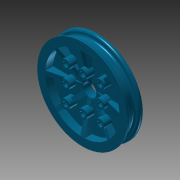
# Autodesk Inventor part: 13-0001
Saved by Autodesk Inventor 2015 SP1 (Build 190203100, 203)
## iProperties
Category: Matrix
Company: Autodesk Inc.
Created: 2014-11-30
Part Number: 13-0001
Material: Polystyrene, High Impact
Document SubType Name: Modeling
Designer: Matrix
Density: 1.022 g/cm^3
Appearance: Sky Blue Dark
Catalog Web Link: http://matrixrobotics.com/
Vendor: Matrix
Author: Autodesk Inc.
Autodesk Inventor part; units mm, degrees
ref_plane "YZ Plane" through (0, 0, 0) normal (1, 0, 0) x (0, 1, 0)
ref_plane "XZ Plane" through (0, 0, 0) normal (0, 1, 0) x (-1, 0, 0)
ref_plane "XY Plane" through (0, 0, 0) normal (0, 0, 1) x (1, 0, 0)
sketch "Sketch1" plane through (0, 0, 0) normal (0, 1, 0) x (-1, 0, 0)
  circle A0 centre (0, 16) radius 2.3444
  circle A1 centre (16, 16) radius 2.3444
  arc A2 (34.4298, 2.2) -> (25.7684, 22.9399) centre (0, 0) ccw
  line L0 (25.7684, 22.9399) -> (25.7597, 22.9313)
  line L1 (25.7597, 22.9313) -> (22.7899, 25.9012)
  arc A3 (22.7899, 25.9012) -> (2, 34.442) centre (0, 0) ccw
  line L2 (2, 34.442) -> (2, 34.4298)
  line L3 (2, 34.4298) -> (-2.2, 34.4298)
  arc A4 (-2.2, 34.4298) -> (-22.9399, 25.7684) centre (0, 0) ccw
  line L4 (-22.9399, 25.7684) -> (-22.9313, 25.7597)
  line L5 (-22.9313, 25.7597) -> (-25.9012, 22.7899)
  arc A5 (-25.9012, 22.7899) -> (-34.442, 2) centre (0, 0) ccw
  line L6 (-34.442, 2) -> (-34.4298, 2)
  line L7 (-34.4298, 2) -> (-34.4298, -2.2)
  arc A6 (-34.4298, -2.2) -> (-25.7684, -22.9399) centre (0, 0) ccw
  line L8 (-25.7684, -22.9399) -> (-25.7597, -22.9313)
  line L9 (-25.7597, -22.9313) -> (-22.7899, -25.9012)
  arc A7 (-22.7899, -25.9012) -> (-2, -34.442) centre (0, 0) ccw
  line L10 (-2, -34.442) -> (-2, -34.4298)
  line L11 (-2, -34.4298) -> (2.2, -34.4298)
  arc A8 (2.2, -34.4298) -> (22.9399, -25.7684) centre (0, 0) ccw
  line L12 (22.9399, -25.7684) -> (22.9313, -25.7597)
  line L13 (22.9313, -25.7597) -> (25.9012, -22.7899)
  arc A9 (25.9012, -22.7899) -> (34.442, -2) centre (0, 0) ccw
  line L14 (34.442, -2) -> (34.4298, -2)
  line L15 (34.4298, -2) -> (34.4298, 2.2)
  circle A10 centre (16, -16) radius 4.265
  circle A11 centre (16, 16) radius 4.265
  circle A12 centre (16, 0) radius 4.265
  circle A13 centre (0, 16) radius 4.265
  circle A14 centre (0, 0) radius 42
  circle A15 centre (0, -16) radius 2.3444
  circle A16 centre (16, -16) radius 2.3444
  circle A17 centre (16, 0) radius 2.3444
  circle A18 centre (-16, 0) radius 4.265
  circle A19 centre (0, -16) radius 4.265
  circle A20 centre (-16, -16) radius 4.265
  circle A21 centre (-16, 16) radius 4.265
  circle A22 centre (-16, -16) radius 2.3444
  circle A23 centre (-16, 0) radius 2.3444
  circle A24 centre (-16, 16) radius 2.3444
  point P0 (0, 0)
  point P1 (0, 0)
  constraints: 32 end point, 25 centre point, 16 point on circle
extrude "Extrusion1" add sketch "Sketch1" along normal blind 14 contours L15 L14 A9 L13 L12 A8 L11 L10 A7 L9 L8 A6 L7 L6 A5 L5 L4 A4 L3 L2 A3 L1 L0 A2 | A10 | A11 | A12 | A13 | A14 | A18 | A19 | A20 | A21
sketch "Sketch2" plane through (0, 0, 0) normal (1, 0, 0) x (0, 1, 0)
  line L0 (14, -13.6556) -> (0, -13.6556) projected
  line L1 (0, -13.6556) -> (0, 13.6556) projected
  line L2 (0, 13.6556) -> (14, 13.6556) projected
  line L3 (14, 13.6556) -> (14, -13.6556) projected
  line L4 (14, -42) -> (0, -42) projected
  line L5 (0, -42) -> (0, -18.3444) projected
  line L6 (0, -18.3444) -> (14, -18.3444) projected
  line L7 (14, -18.3444) -> (14, -42) projected
  line L8 (0, 42) -> (14, 42) projected
  line L9 (14, 42) -> (14, 18.3444) projected
  line L10 (14, 18.3444) -> (0, 18.3444) projected
  line L11 (0, 18.3444) -> (0, 42) projected
  line L12 (0, 42) -> (1, 42)
  arc A0 (3, 40) -> (1, 42) centre (1, 40) ccw
  line L13 (3, 40) -> (3, 39.5)
  arc A1 (3, 39.5) -> (5, 37.5) centre (5, 39.5) ccw
  line L14 (5, 37.5) -> (9, 37.5)
  arc A2 (9, 37.5) -> (11, 39.5) centre (9, 39.5) ccw
  line L15 (11, 39.5) -> (11, 40)
  arc A3 (13, 42) -> (11, 40) centre (13, 40) ccw
  line L16 (13, 42) -> (14, 42)
  line L17 (14, 42) -> (14, 40)
  line L18 (14, 40) -> (13, 39.9913)
  line L19 (13, 39.9913) -> (13, 39.0087)
  line L20 (13, 39.0087) -> (14, 39)
  line L21 (14, 39) -> (14, 37.0133)
  line L22 (1, 42) -> (13, 42)
  line L23 (14, 40) -> (14, 39)
  line L24 (-2.8, 0) -> (16.8, 0) projected
  point P0 (0, 0)
  constraints: 24 end point, 8 point on circle, 4 centre point, 1 collinear, 1 vertical
revolve "Revolution1" cut sketch "Sketch2" angle 360 about axis through (0, -10, 0) along (0, 1, 0) contours L8 A3 L15 A2 L14 A1 L13 A0 | L9 L20 L19 L18
sketch "Sketch3" plane through (0, 14, 0) normal (0, 1, 0) x (1, 0, 0)
  arc A0 (-24.8311, -28.7649) -> (-2.7753, -37.8985) centre (0, 0) ccw
  line L0 (-2.7753, -37.8985) -> (-2.7753, -6.7092)
  line L1 (-2.7753, -6.7092) -> (-24.8311, -28.7649)
  line L2 (14.3804, 14.6632) -> (4.8177, 5.1006)
  line L3 (4.8177, 5.1006) -> (5.1006, 4.8177)
  line L4 (5.1006, 4.8177) -> (14.6632, 14.3804)
  arc A1 (14.6632, 14.3804) -> (15.1927, 14.0614) centre (16, 16) ccw
  line L5 (15.1927, 14.0614) -> (5.5248, 4.3934)
  line L6 (5.5248, 4.3934) -> (5.8077, 4.1106)
  line L7 (5.8077, 4.1106) -> (15.6299, 13.9329)
  arc A2 (15.6299, 13.9329) -> (18.0671, 16.3701) centre (16, 16) ccw
  line L8 (18.0671, 16.3701) -> (27.0209, 25.3238)
  line L9 (27.0209, 25.3238) -> (26.738, 25.6066)
  line L10 (26.738, 25.6066) -> (17.9386, 16.8073)
  arc A3 (17.9386, 16.8073) -> (17.6196, 17.3368) centre (16, 16) ccw
  line L11 (17.6196, 17.3368) -> (26.3138, 26.0309)
  line L12 (26.3138, 26.0309) -> (26.0309, 26.3138)
  line L13 (26.0309, 26.3138) -> (17.3368, 17.6196)
  arc A4 (17.3368, 17.6196) -> (16.8073, 17.9386) centre (16, 16) ccw
  line L14 (16.8073, 17.9386) -> (25.6066, 26.738)
  line L15 (25.6066, 26.738) -> (25.3238, 27.0209)
  line L16 (25.3238, 27.0209) -> (16.3701, 18.0671)
  arc A5 (16.3701, 18.0671) -> (13.9329, 15.6299) centre (16, 16) ccw
  line L17 (13.9329, 15.6299) -> (4.1106, 5.8077)
  line L18 (4.1106, 5.8077) -> (4.3934, 5.5248)
  line L19 (4.3934, 5.5248) -> (14.0614, 15.1927)
  arc A6 (14.0614, 15.1927) -> (14.3804, 14.6632) centre (16, 16) ccw
  line L20 (7.0133, 1.2) -> (7.0133, 0.8)
  line L21 (7.0133, 0.8) -> (14.0584, 0.8)
  arc A7 (14.0584, 0.8) -> (13.9095, 0.2) centre (16, 0) ccw
  line L22 (13.9095, 0.2) -> (7.0133, 0.2)
  line L23 (7.0133, 0.2) -> (7.0133, -0.2)
  line L24 (7.0133, -0.2) -> (13.9095, -0.2)
  arc A8 (13.9095, -0.2) -> (14.0584, -0.8) centre (16, 0) ccw
  line L25 (14.0584, -0.8) -> (7.0133, -0.8)
  line L26 (7.0133, -0.8) -> (7.0133, -1.2)
  line L27 (7.0133, -1.2) -> (14.2766, -1.2)
  arc A9 (14.2766, -1.2) -> (17.7234, -1.2) centre (16, 0) ccw
  line L28 (17.7234, -1.2) -> (37.0133, -1.2)
  line L29 (37.0133, -1.2) -> (37.0133, -0.8)
  line L30 (37.0133, -0.8) -> (17.9416, -0.8)
  arc A10 (17.9416, -0.8) -> (18.0905, -0.2) centre (16, 0) ccw
  line L31 (18.0905, -0.2) -> (37.0133, -0.2)
  line L32 (37.0133, -0.2) -> (37.0133, 0.2)
  line L33 (37.0133, 0.2) -> (18.0905, 0.2)
  arc A11 (18.0905, 0.2) -> (17.9416, 0.8) centre (16, 0) ccw
  line L34 (17.9416, 0.8) -> (37.0133, 0.8)
  line L35 (37.0133, 0.8) -> (37.0133, 1.2)
  line L36 (37.0133, 1.2) -> (17.7234, 1.2)
  arc A12 (17.7234, 1.2) -> (14.2766, 1.2) centre (16, 0) ccw
  line L37 (14.2766, 1.2) -> (7.0133, 1.2)
  line L38 (5.8077, -4.1106) -> (5.5248, -4.3934)
  line L39 (5.5248, -4.3934) -> (15.1927, -14.0614)
  arc A13 (15.1927, -14.0614) -> (14.6632, -14.3804) centre (16, -16) ccw
  line L40 (14.6632, -14.3804) -> (5.1006, -4.8177)
  line L41 (5.1006, -4.8177) -> (4.8177, -5.1006)
  line L42 (4.8177, -5.1006) -> (14.3804, -14.6632)
  arc A14 (14.3804, -14.6632) -> (14.0614, -15.1927) centre (16, -16) ccw
  line L43 (14.0614, -15.1927) -> (4.3934, -5.5248)
  line L44 (4.3934, -5.5248) -> (4.1106, -5.8077)
  line L45 (4.1106, -5.8077) -> (13.9329, -15.6299)
  arc A15 (13.9329, -15.6299) -> (16.3701, -18.0671) centre (16, -16) ccw
  line L46 (16.3701, -18.0671) -> (25.3238, -27.0209)
  line L47 (25.3238, -27.0209) -> (25.6066, -26.738)
  line L48 (25.6066, -26.738) -> (16.8073, -17.9386)
  arc A16 (16.8073, -17.9386) -> (17.3368, -17.6196) centre (16, -16) ccw
  line L49 (17.3368, -17.6196) -> (26.0309, -26.3138)
  line L50 (26.0309, -26.3138) -> (26.3138, -26.0309)
  line L51 (26.3138, -26.0309) -> (17.6196, -17.3368)
  arc A17 (17.6196, -17.3368) -> (17.9386, -16.8073) centre (16, -16) ccw
  line L52 (17.9386, -16.8073) -> (26.738, -25.6066)
  line L53 (26.738, -25.6066) -> (27.0209, -25.3238)
  line L54 (27.0209, -25.3238) -> (18.0671, -16.3701)
  arc A18 (18.0671, -16.3701) -> (15.6299, -13.9329) centre (16, -16) ccw
  line L55 (15.6299, -13.9329) -> (5.8077, -4.1106)
  line L56 (-5.8077, 4.1106) -> (-5.5248, 4.3934)
  line L57 (-5.5248, 4.3934) -> (-15.1927, 14.0614)
  arc A19 (-15.1927, 14.0614) -> (-14.6632, 14.3804) centre (-16, 16) ccw
  line L58 (-14.6632, 14.3804) -> (-5.1006, 4.8177)
  line L59 (-5.1006, 4.8177) -> (-4.8177, 5.1006)
  line L60 (-4.8177, 5.1006) -> (-14.3804, 14.6632)
  arc A20 (-14.3804, 14.6632) -> (-14.0614, 15.1927) centre (-16, 16) ccw
  line L61 (-14.0614, 15.1927) -> (-4.3934, 5.5248)
  line L62 (-4.3934, 5.5248) -> (-4.1106, 5.8077)
  line L63 (-4.1106, 5.8077) -> (-13.9329, 15.6299)
  arc A21 (-13.9329, 15.6299) -> (-16.3701, 18.0671) centre (-16, 16) ccw
  line L64 (-16.3701, 18.0671) -> (-25.3238, 27.0209)
  line L65 (-25.3238, 27.0209) -> (-25.6066, 26.738)
  line L66 (-25.6066, 26.738) -> (-16.8073, 17.9386)
  arc A22 (-16.8073, 17.9386) -> (-17.3368, 17.6196) centre (-16, 16) ccw
  line L67 (-17.3368, 17.6196) -> (-26.0309, 26.3138)
  line L68 (-26.0309, 26.3138) -> (-26.3138, 26.0309)
  line L69 (-26.3138, 26.0309) -> (-17.6196, 17.3368)
  arc A23 (-17.6196, 17.3368) -> (-17.9386, 16.8073) centre (-16, 16) ccw
  line L70 (-17.9386, 16.8073) -> (-26.738, 25.6066)
  line L71 (-26.738, 25.6066) -> (-27.0209, 25.3238)
  line L72 (-27.0209, 25.3238) -> (-18.0671, 16.3701)
  arc A24 (-18.0671, 16.3701) -> (-15.6299, 13.9329) centre (-16, 16) ccw
  line L73 (-15.6299, 13.9329) -> (-5.8077, 4.1106)
  line L74 (0.8, 7.0133) -> (1.2, 7.0133)
  line L75 (1.2, 7.0133) -> (1.2, 14.2766)
  arc A25 (1.2, 14.2766) -> (1.2, 17.7234) centre (0, 16) ccw
  line L76 (1.2, 17.7234) -> (1.2, 37.0133)
  line L77 (1.2, 37.0133) -> (0.8, 37.0133)
  line L78 (0.8, 37.0133) -> (0.8, 17.9416)
  arc A26 (0.8, 17.9416) -> (0.2, 18.0905) centre (0, 16) ccw
  line L79 (0.2, 18.0905) -> (0.2, 37.0133)
  line L80 (0.2, 37.0133) -> (-0.2, 37.0133)
  line L81 (-0.2, 37.0133) -> (-0.2, 18.0905)
  arc A27 (-0.2, 18.0905) -> (-0.8, 17.9416) centre (0, 16) ccw
  line L82 (-0.8, 17.9416) -> (-0.8, 37.0133)
  line L83 (-0.8, 37.0133) -> (-1.2, 37.0133)
  line L84 (-1.2, 37.0133) -> (-1.2, 17.7234)
  arc A28 (-1.2, 17.7234) -> (-1.2, 14.2766) centre (0, 16) ccw
  line L85 (-1.2, 14.2766) -> (-1.2, 7.0133)
  line L86 (-1.2, 7.0133) -> (-0.8, 7.0133)
  line L87 (-0.8, 7.0133) -> (-0.8, 14.0584)
  arc A29 (-0.8, 14.0584) -> (-0.2, 13.9095) centre (0, 16) ccw
  line L88 (-0.2, 13.9095) -> (-0.2, 7.0133)
  line L89 (-0.2, 7.0133) -> (0.2, 7.0133)
  line L90 (0.2, 7.0133) -> (0.2, 13.9095)
  arc A30 (0.2, 13.9095) -> (0.8, 14.0584) centre (0, 16) ccw
  line L91 (0.8, 14.0584) -> (0.8, 7.0133)
  line L92 (-6.7065, -2.7816) -> (-37.8981, -2.7816)
  arc A31 (-37.8981, -2.7816) -> (-28.7608, -24.8358) centre (0, 0) ccw
  line L93 (-28.7608, -24.8358) -> (-6.7065, -2.7816)
  line L94 (-2.7816, 6.7065) -> (-2.7816, 37.8981)
  arc A32 (-2.7816, 37.8981) -> (-24.8358, 28.7608) centre (0, 0) ccw
  line L95 (-24.8358, 28.7608) -> (-2.7816, 6.7065)
  line L96 (2.7753, 6.7092) -> (24.8311, 28.7649)
  arc A33 (24.8311, 28.7649) -> (2.7753, 37.8985) centre (0, 0) ccw
  line L97 (2.7753, 37.8985) -> (2.7753, 6.7092)
  line L98 (6.7065, 2.7816) -> (37.8981, 2.7816)
  arc A34 (37.8981, 2.7816) -> (28.7608, 24.8358) centre (0, 0) ccw
  line L99 (28.7608, 24.8358) -> (6.7065, 2.7816)
  line L100 (6.7092, -2.7753) -> (28.7649, -24.8311)
  arc A35 (28.7649, -24.8311) -> (37.8985, -2.7753) centre (0, 0) ccw
  line L101 (37.8985, -2.7753) -> (6.7092, -2.7753)
  line L102 (2.7816, -6.7065) -> (2.7816, -37.8981)
  arc A36 (2.7816, -37.8981) -> (24.8358, -28.7608) centre (0, 0) ccw
  line L103 (24.8358, -28.7608) -> (2.7816, -6.7065)
  line L104 (-6.7092, 2.7753) -> (-28.7649, 24.8311)
  arc A37 (-28.7649, 24.8311) -> (-37.8985, 2.7753) centre (0, 0) ccw
  line L105 (-37.8985, 2.7753) -> (-6.7092, 2.7753)
  circle A38 centre (0, 0) radius 40
  circle A39 centre (0, 0) radius 39
  line L106 (1.2, -7.0133) -> (0.8, -7.0133)
  line L107 (0.8, -7.0133) -> (0.8, -14.0584)
  arc A40 (0.8, -14.0584) -> (0.2, -13.9095) centre (0, -16) ccw
  line L108 (0.2, -13.9095) -> (0.2, -7.0133)
  line L109 (0.2, -7.0133) -> (-0.2, -7.0133)
  line L110 (-0.2, -7.0133) -> (-0.2, -13.9095)
  arc A41 (-0.2, -13.9095) -> (-0.8, -14.0584) centre (0, -16) ccw
  line L111 (-0.8, -14.0584) -> (-0.8, -7.0133)
  line L112 (-0.8, -7.0133) -> (-1.2, -7.0133)
  line L113 (-1.2, -7.0133) -> (-1.2, -14.2766)
  arc A42 (-1.2, -14.2766) -> (-1.2, -17.7234) centre (0, -16) ccw
  line L114 (-1.2, -17.7234) -> (-1.2, -37.0133)
  line L115 (-1.2, -37.0133) -> (-0.8, -37.0133)
  line L116 (-0.8, -37.0133) -> (-0.8, -17.9416)
  arc A43 (-0.8, -17.9416) -> (-0.2, -18.0905) centre (0, -16) ccw
  line L117 (-0.2, -18.0905) -> (-0.2, -37.0133)
  line L118 (-0.2, -37.0133) -> (0.2, -37.0133)
  line L119 (0.2, -37.0133) -> (0.2, -18.0905)
  arc A44 (0.2, -18.0905) -> (0.8, -17.9416) centre (0, -16) ccw
  line L120 (0.8, -17.9416) -> (0.8, -37.0133)
  line L121 (0.8, -37.0133) -> (1.2, -37.0133)
  line L122 (1.2, -37.0133) -> (1.2, -17.7234)
  arc A45 (1.2, -17.7234) -> (1.2, -14.2766) centre (0, -16) ccw
  line L123 (1.2, -14.2766) -> (1.2, -7.0133)
  line L124 (-4.1106, -5.8077) -> (-4.3934, -5.5248)
  line L125 (-4.3934, -5.5248) -> (-14.0614, -15.1927)
  arc A46 (-14.0614, -15.1927) -> (-14.3804, -14.6632) centre (-16, -16) ccw
  line L126 (-14.3804, -14.6632) -> (-4.8177, -5.1006)
  line L127 (-4.8177, -5.1006) -> (-5.1006, -4.8177)
  line L128 (-5.1006, -4.8177) -> (-14.6632, -14.3804)
  arc A47 (-14.6632, -14.3804) -> (-15.1927, -14.0614) centre (-16, -16) ccw
  line L129 (-15.1927, -14.0614) -> (-5.5248, -4.3934)
  line L130 (-5.5248, -4.3934) -> (-5.8077, -4.1106)
  line L131 (-5.8077, -4.1106) -> (-15.6299, -13.9329)
  arc A48 (-15.6299, -13.9329) -> (-18.0671, -16.3701) centre (-16, -16) ccw
  line L132 (-18.0671, -16.3701) -> (-27.0209, -25.3238)
  line L133 (-27.0209, -25.3238) -> (-26.738, -25.6066)
  line L134 (-26.738, -25.6066) -> (-17.9386, -16.8073)
  arc A49 (-17.9386, -16.8073) -> (-17.6196, -17.3368) centre (-16, -16) ccw
  line L135 (-17.6196, -17.3368) -> (-26.3138, -26.0309)
  line L136 (-26.3138, -26.0309) -> (-26.0309, -26.3138)
  line L137 (-26.0309, -26.3138) -> (-17.3368, -17.6196)
  arc A50 (-17.3368, -17.6196) -> (-16.8073, -17.9386) centre (-16, -16) ccw
  line L138 (-16.8073, -17.9386) -> (-25.6066, -26.738)
  line L139 (-25.6066, -26.738) -> (-25.3238, -27.0209)
  line L140 (-25.3238, -27.0209) -> (-16.3701, -18.0671)
  arc A51 (-16.3701, -18.0671) -> (-13.9329, -15.6299) centre (-16, -16) ccw
  line L141 (-13.9329, -15.6299) -> (-4.1106, -5.8077)
  circle A52 centre (0, 0) radius 42
  circle A53 centre (0, 0) radius 6
  line L142 (-7.0133, 0.8) -> (-7.0133, 1.2)
  line L143 (-7.0133, 1.2) -> (-14.2766, 1.2)
  arc A54 (-14.2766, 1.2) -> (-17.7234, 1.2) centre (-16, 0) ccw
  line L144 (-17.7234, 1.2) -> (-37.0133, 1.2)
  line L145 (-37.0133, 1.2) -> (-37.0133, 0.8)
  line L146 (-37.0133, 0.8) -> (-17.9416, 0.8)
  arc A55 (-17.9416, 0.8) -> (-18.0905, 0.2) centre (-16, 0) ccw
  line L147 (-18.0905, 0.2) -> (-37.0133, 0.2)
  line L148 (-37.0133, 0.2) -> (-37.0133, -0.2)
  line L149 (-37.0133, -0.2) -> (-18.0905, -0.2)
  arc A56 (-18.0905, -0.2) -> (-17.9416, -0.8) centre (-16, 0) ccw
  line L150 (-17.9416, -0.8) -> (-37.0133, -0.8)
  line L151 (-37.0133, -0.8) -> (-37.0133, -1.2)
  line L152 (-37.0133, -1.2) -> (-17.7234, -1.2)
  arc A57 (-17.7234, -1.2) -> (-14.2766, -1.2) centre (-16, 0) ccw
  line L153 (-14.2766, -1.2) -> (-7.0133, -1.2)
  line L154 (-7.0133, -1.2) -> (-7.0133, -0.8)
  line L155 (-7.0133, -0.8) -> (-14.0584, -0.8)
  arc A58 (-14.0584, -0.8) -> (-13.9095, -0.2) centre (-16, 0) ccw
  line L156 (-13.9095, -0.2) -> (-7.0133, -0.2)
  line L157 (-7.0133, -0.2) -> (-7.0133, 0.2)
  line L158 (-7.0133, 0.2) -> (-13.9095, 0.2)
  arc A59 (-13.9095, 0.2) -> (-14.0584, 0.8) centre (-16, 0) ccw
  line L159 (-14.0584, 0.8) -> (-7.0133, 0.8)
  point P0 (0, 0)
  constraints: 320 end point, 112 point on circle, 60 centre point
extrude "Extrusion2" cut sketch "Sketch3" against normal blind 2 contours L1 L0 A0 | L93 A31 L92 | L95 A32 L94 | L97 A33 L96 | L99 A34 L98 | L101 A35 L100 | L103 A36 L102 | L105 A37 L104
extrude "Extrusion3" cut sketch "Sketch1" along normal blind 7 contours L15 L14 A9 L13 L12 A8 L11 L10 A7 L9 L8 A6 L7 L6 A5 L5 L4 A4 L3 L2 A3 L1 L0 A2
sketch "Sketch5" plane through (0, 14, 0) normal (0, 1, 0) x (1, 0, 0)
  point P0 (0, 0)
hole "Hole1" at (0, 14, 0) direction (0, -1, 0) diameter 12 end through all
sketch "Sketch6" plane through (0, 0, 0) normal (1, 0, 0) x (0, 1, 0)
  line L0 (7, 11.735) -> (0, 11.735) projected
  line L1 (0, 11.735) -> (0, 13.6556) projected
  line L2 (0, 13.6556) -> (14, 13.6556) projected
  line L3 (14, 13.6556) -> (14, 6) projected
  line L4 (14, 6) -> (7, 6) projected
  line L5 (7, 6) -> (7, 11.735) projected
  line L6 (0, -11.735) -> (7, -11.735) projected
  line L7 (7, -11.735) -> (7, -6) projected
  line L8 (7, -6) -> (14, -6) projected
  line L9 (14, -6) -> (14, -13.6556) projected
  line L10 (14, -13.6556) -> (0, -13.6556) projected
  line L11 (0, -13.6556) -> (0, -11.735) projected
  line L12 (3, 40) -> (3, 39.5) projected
  arc A0 (3, 39.5) -> (5, 37.5) centre (5, 39.5) ccw projected
  line L13 (5, 37.5) -> (9, 37.5) projected
  arc A1 (9, 37.5) -> (11, 39.5) centre (9, 39.5) ccw projected
  line L14 (11, 39.5) -> (11, 40) projected
  arc A2 (13, 42) -> (11, 40) centre (13, 40) ccw projected
  line L15 (13, 42) -> (14, 42) projected
  line L16 (14, 42) -> (14, 40) projected
  line L17 (14, 40) -> (13, 39.9913) projected
  line L18 (13, 39.9913) -> (13, 39.0087) projected
  line L19 (13, 39.0087) -> (14, 39) projected
  line L20 (14, 39) -> (14, 18.3444) projected
  line L21 (14, 18.3444) -> (0, 18.3444) projected
  line L22 (0, 18.3444) -> (0, 20.265) projected
  line L23 (0, 20.265) -> (7, 20.265) projected
  line L24 (7, 20.265) -> (7, 34.4298) projected
  line L25 (7, 34.4298) -> (0, 34.4298) projected
  line L26 (0, 34.4298) -> (0, 42) projected
  line L27 (0, 42) -> (1, 42) projected
  arc A3 (3, 40) -> (1, 42) centre (1, 40) ccw projected
  line L28 (3, -39.5) -> (3, -40) projected
  arc A4 (1, -42) -> (3, -40) centre (1, -40) ccw projected
  line L29 (1, -42) -> (0, -42) projected
  line L30 (0, -42) -> (0, -34.4298) projected
  line L31 (0, -34.4298) -> (7, -34.4298) projected
  line L32 (7, -34.4298) -> (7, -20.265) projected
  line L33 (7, -20.265) -> (0, -20.265) projected
  line L34 (0, -20.265) -> (0, -18.3444) projected
  line L35 (0, -18.3444) -> (14, -18.3444) projected
  line L36 (14, -18.3444) -> (14, -39) projected
  line L37 (14, -39) -> (13, -39.0087) projected
  line L38 (13, -39.0087) -> (13, -39.9913) projected
  line L39 (13, -39.9913) -> (14, -40) projected
  line L40 (14, -40) -> (14, -42) projected
  line L41 (14, -42) -> (13, -42) projected
  arc A5 (11, -40) -> (13, -42) centre (13, -40) ccw projected
  line L42 (11, -40) -> (11, -39.5) projected
  arc A6 (11, -39.5) -> (9, -37.5) centre (9, -39.5) ccw projected
  line L43 (9, -37.5) -> (5, -37.5) projected
  arc A7 (5, -37.5) -> (3, -39.5) centre (5, -39.5) ccw projected
  line L44 (0, 34.4298) -> (7, 6)
  line L45 (0, 34.4298) -> (7, 34.4298)
  line L46 (14, 37.8985) -> (14, 28.7649) projected
  line L47 (7, 6) -> (7, 34.4298)
  line L48 (14, -39) -> (14, 39) projected
  point P0 (0, 0)
  constraints: 6 end point, 1 perpendicular, 1 vertical, 1 other
extrude "Extrusion4" add sketch "Sketch6" along normal mid plane 4 contours L5 L44 L0 | L0 L44 L2 L47 | L2 L44 L21 L47 | L21 L44 L23 L47 | L23 L44 L25 L24
pattern_circular "Circular Pattern1" count 8 over 360 about axis through (0, -105.6161, 0) along (0, 1, 0) of "Extrusion4"
body "Solid1"
